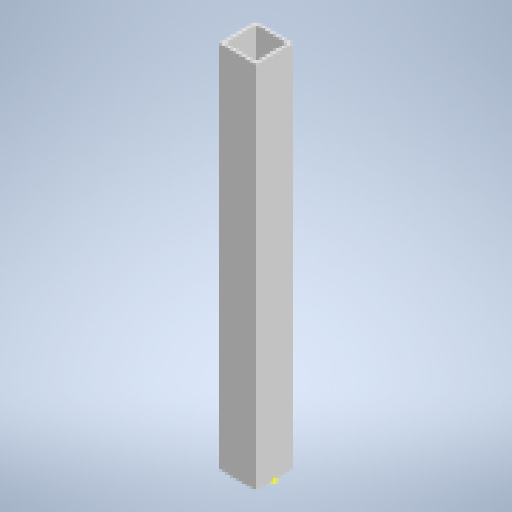
# Autodesk Inventor part: Tube 40 cm
Saved by Autodesk Inventor 2025 (Build 290162000, 162)
## iProperties
Created: 2024-06-27
Part Number: Tube 40 cm
Material: Generic
Document SubType Name: Modeling
Designer: User
Density: 1 g/cm^3
Appearance: Default
Author: User
Autodesk Inventor part; units mm, degrees
ref_plane "YZ Plane" through (0, 0, 0) normal (1, 0, 0) x (0, 1, 0)
ref_plane "XZ Plane" through (0, 0, 0) normal (0, 1, 0) x (-1, 0, 0)
ref_plane "XY Plane" through (0, 0, 0) normal (0, 0, 1) x (1, 0, 0)
sketch "Sketch1" plane through (0, 0, 0) normal (0, 1, 0) x (-1, 0, 0)
  line L0 (-20, 20) -> (20, 20)
  line L1 (20, 20) -> (20, -20)
  line L2 (20, -20) -> (-20, -20)
  line L3 (-20, -20) -> (-20, 20)
  line L4 (-20, 20) -> (20, -20) construction
  line L5 (20, 20) -> (-20, -20) construction
  line L6 (-17, 17) -> (17, 17)
  line L7 (17, 17) -> (17, -17)
  line L8 (17, -17) -> (-17, -17)
  line L9 (-17, -17) -> (-17, 17)
  line L10 (-17, 17) -> (17, -17) construction
  line L11 (17, 17) -> (-17, -17) construction
  point P0 (0, 0)
  dimension "d0" = 40
  dimension "d1" = 40
  dimension "d2" = 34
  dimension "d3" = 34
  dimension "d4" = 3
  constraints: 24 end point, 4 midpoint, 4 parallel, 2 horizontal, 2 perpendicular
  measures "d0" distance of L0.end L1.end
  measures "d1" distance of L1.end L2.end
  measures "d2" distance of L7.end L8.end
  measures "d3" distance of L6.end L7.end
  measures "d4" distance between parallel lines of L7 L1
extrude "Extrusion1" add sketch "Sketch1" along normal blind 390
sketch "Sketch2" plane through (20, 0, 20) normal (1, 0, 0) x (0, 0, -1)
  point P0 (20, 0)
body "Solid1"
